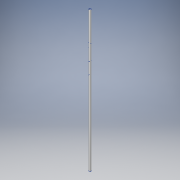
# Autodesk Inventor part: tubo_instrumentação_2500mm
Saved by Autodesk Inventor 2019.4 (Build 234330000, 330)
## iProperties
Created: 2021-02-17
Part Number: tubo_instrumentação_2500mm
Material: Alumínio 6061
Document SubType Name: Modeling
Designer: Lattes
Density: 2.7 g/cm^3
Appearance: Alumínio - Plano
Author: Lattes
Autodesk Inventor part; units mm, degrees
ref_plane "XZ Plane" through (0, 0, 0) normal (0, 1, 0) x (-1, 0, 0)
sketch "Esboço1" plane through (0, 0, 0) normal (0, 1, 0) x (-1, 0, 0)
  circle A0 centre (0, 0) radius 14.5
  circle A1 centre (0, 0) radius 16
  dimension "d0" = 29
  dimension "d1" = 32
  constraints: 2 centre point, 2 coincident
  measures "d0" diameter of A0
  measures "d1" diameter of A1
extrude "Extrusão1" add sketch "Esboço1" along normal blind 2500
ref_plane "Plano de trabalho2" through (-16, 0, 0) normal (1, 0, 0) x (0, 1, 0)
sketch "Esboço2" plane through (-16, 0, 0) normal (1, 0, 0) x (0, 1, 0)
  line L0 (2500, -16) -> (2500, 16) projected
  line L1 (2500, 0) -> (1900, 0)
  circle A0 centre (1900, 0) radius 1.75
  circle A1 centre (1900, 0) radius 3
  point P0 (0, 0)
  dimension "d6" = 600
  dimension "d7" = 3.5
  dimension "d8" = 6
  constraints: 2 centre point, 2 coincident, 2 end point, 1 horizontal, 1 midpoint
  measures "d6" distance of L1.start L1.end
  measures "d7" diameter of A0
  measures "d8" diameter of A1
extrude "Extrusão2" add sketch "Esboço2" along normal blind 0.5
sketch "Esboço3" plane through (-16, 0, 0) normal (-1, 0, 0) x (0, 0, 1)
  arc A0 (0, 1898.25) -> (0, 1901.75) centre (0, 1900) ccw projected
  circle A1 centre (0, 1900) radius 1.75
  point P0 (0, 0)
  constraints: 1 centre point, 1 coincident
extrude "Extrusão3" cut sketch "Esboço3" against normal blind 5
sketch "Esboço4" plane through (-16, 0, 0) normal (1, 0, 0) x (0, 1, 0)
  line L0 (2500, 14.5) -> (2500, -14.5) projected
  line L1 (2500, 0) -> (1840, 0)
  line L2 (1840, 0) -> (1470, 0)
  circle A0 centre (1470, 0) radius 1.75
  circle A1 centre (1470, 0) radius 3
  line L3 (1470, 0) -> (1430, 0)
  line L4 (1470, 0) -> (1510, 0) construction
  point P0 (0, 0)
  dimension "d13" = 660
  dimension "d14" = 370
  dimension "d15" = 3.5
  dimension "d16" = 6
  dimension "d21" = 40
  dimension "d22" = 180
  constraints: 8 end point, 3 horizontal, 2 centre point, 2 coincident, 1 collinear, 1 midpoint, 1 point on line
  measures "d13" distance of L1.start L1.end
  measures "d14" distance of L1.end L2.end
  measures "d15" diameter of A0
  measures "d16" diameter of A1
  measures "d21" distance of L3.start L3.end
  measures "d22" angle of L3 L4
extrude "Extrusão4" add sketch "Esboço4" along normal blind 0.5 contours A1 L3 A0 L2 | L2 A0 L3 A1
sketch "Esboço5" plane through (-16, 0, 0) normal (-1, 0, 0) x (0, 0, 1)
  arc A0 (0, 1468.25) -> (0, 1471.75) centre (0, 1470) ccw projected
  circle A1 centre (0, 1470) radius 1.75
  point P0 (0, 0)
  point P1 (0, 1741.75)
  point P2 (0, 1738.25)
  point P3 (0, 1438.25)
  point P4 (0, 1441.75)
  constraints: 1 coincident, 3 other
extrude "Extrusão5" cut sketch "Esboço5" against normal blind 4
ref_plane "Plano de trabalho3" through (0, 0, 16) normal (0, 0, 1) x (1, 0, 0)
sketch "Esboço6" plane through (0, 0, 16) normal (0, 0, 1) x (1, 0, 0)
  line L0 (16, 2500) -> (-16, 2500) projected
  line L1 (0, 2500) -> (0, 1500)
  line L2 (0, 2500) -> (1000, 2500) construction
  circle A0 centre (0, 1500) radius 1.5
  circle A1 centre (0, 1500) radius 3
  point P0 (0, 0)
  dimension "d24" = 1000
  dimension "d25" = 90
  dimension "d26" = 3
  dimension "d27" = 6
  constraints: 4 end point, 2 centre point, 2 coincident, 1 horizontal, 1 midpoint, 1 perpendicular, 1 vertical
  measures "d24" distance of L1.start L1.end
  measures "d25" angle of L1 L2
  measures "d26" diameter of A0
  measures "d27" diameter of A1
extrude "Extrusão6" add sketch "Esboço6" against normal blind 0.4
sketch "Esboço7" plane through (0, 0, 16) normal (0, 0, 1) x (1, 0, 0)
  arc A0 (0, 1498.5) -> (0, 1501.5) centre (0, 1500) ccw projected
  circle A1 centre (0, 1500) radius 1.5
  point P0 (0, 0)
  dimension "d30" = 3
  constraints: 1 centre point, 1 coincident
  measures "d30" diameter of A1
extrude "Extrusão7" cut sketch "Esboço7" against normal blind 10
sketch "Esboço8" plane through (-16, 0, 0) normal (-1, 0, 0) x (0, 0, 1)
  arc A0 (0, 1903) -> (0, 1897) centre (0, 1900) ccw projected
  circle A1 centre (0, 1760) radius 4
  circle A2 centre (0, 1760) radius 3
  line L0 (0, 1760) -> (0, 1840)
  circle A3 centre (0, 1840) radius 3
  circle A4 centre (0, 1840) radius 4
  line L1 (0, 1840) -> (0, 1980)
  circle A5 centre (0, 1980) radius 3
  circle A6 centre (0, 1980) radius 4
  point P0 (0, 0)
  dimension "d34" = 8
  dimension "d35" = 80
  dimension "d36" = 6
  dimension "d37" = 8
  dimension "d38" = 140
  dimension "d39" = 6
  dimension "d40" = 8
  constraints: 6 centre point, 5 coincident, 4 end point, 2 vertical
  measures "d34" diameter of A1
  measures "d35" distance of L0.start L0.end
  measures "d36" diameter of A3
  measures "d37" diameter of A4
  measures "d38" distance of L1.start L1.end
  measures "d39" diameter of A5
  measures "d40" diameter of A6
extrude "Extrusão8" add sketch "Esboço8" against normal blind 0.6 contours A6
sketch "Esboço9" plane through (-16, 0, 0) normal (-1, 0, 0) x (0, 0, 1)
  arc A0 (0, 1977) -> (0, 1983) centre (0, 1980) ccw projected
  circle A1 centre (0, 1980) radius 3
  point P0 (0, 0)
  constraints: 1 centre point, 1 coincident
extrude "Extrusão9" cut sketch "Esboço9" against normal blind 10
pattern_circular "Padrão circular1" count 2 over 360 about axis through (0, -10, 0) along (0, 1, 0) of "Extrusão8"
sketch "Esboço10" plane through (16, 1980, 0) normal (1, 0, 0) x (0, 0, 1)
  circle A0 centre (0, 0) radius 3
  point P0 (0, 1980)
  constraints: 1 centre point
extrude "Extrusão10" cut sketch "Esboço10" against normal blind 10
sketch "Esboço11" plane through (0, 0, 16) normal (0, 0, 1) x (1, 0, 0)
  circle A0 centre (0, 1500) radius 1.5 projected
  line L0 (0, 1500) -> (0, 1700)
  circle A1 centre (0, 1700) radius 3
  circle A2 centre (0, 1700) radius 4
  point P0 (0, 0)
  dimension "d50" = 200
  dimension "d51" = 6
  dimension "d52" = 8
  constraints: 2 centre point, 2 coincident, 2 end point, 1 vertical
  measures "d50" distance of L0.start L0.end
  measures "d51" diameter of A1
  measures "d52" diameter of A2
extrude "Extrusão11" add sketch "Esboço11" against normal blind 0.6 contours A2
pattern_circular "Padrão circular2" count 2 over 360 about axis through (0, -10, 0) along (0, 1, 0) of "Extrusão11"
sketch "Esboço12" plane through (0, 0, 16) normal (0, 0, 1) x (1, 0, 0)
  arc A0 (0, 1703) -> (0, 1697) centre (0, 1700) ccw projected
  circle A1 centre (0, 1700) radius 3
  point P0 (0, 0)
  constraints: 1 centre point, 1 coincident
extrude "Extrusão12" cut sketch "Esboço12" against normal blind 60
